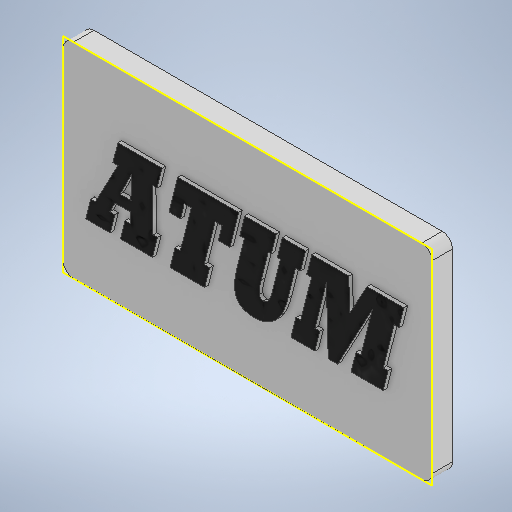
# Autodesk Inventor part: custom plate
Saved by Autodesk Inventor 2025.1 (Build 291241020, 241B)
## iProperties
Created: 2024-12-05
Part Number: custom plate
Material: Generic
Document SubType Name: Modeling
Designer: Hunter Mathis
Density: 1 g/cm^3
Appearance: Default
Author: Hunter Mathis
Autodesk Inventor part; units mm, degrees
ref_plane "YZ Plane" through (0, 0, 0) normal (1, 0, 0) x (0, 1, 0)
ref_plane "XZ Plane" through (0, 0, 0) normal (0, 1, 0) x (-1, 0, 0)
ref_plane "XY Plane" through (0, 0, 0) normal (0, 0, 1) x (1, 0, 0)
sketch "Sketch1" plane through (0, 0, 0) normal (0, 0, 1) x (1, 0, 0)
  line L0 (0, 0) -> (-114.3, 0)
  line L1 (-114.3, 0) -> (-114.3, 63.5)
  line L2 (-114.3, 63.5) -> (0, 63.5)
  line L3 (0, 63.5) -> (0, 0)
  dimension "d7" = 114.3
  dimension "d8" = 63.5
  constraints: 8 end point, 2 parallel, 1 horizontal, 1 perpendicular
  measures "d7" distance of L1.end L2.end
  measures "d8" distance of L0.end L1.end
extrude "Extrusion1" add sketch "Sketch1" along normal blind 6.35
sketch "Sketch2" plane through (0, 0, 6.35) normal (0, 0, 1) x (1, 0, 0)
  line L0 (0, 0) -> (0, 63.5) projected
  line L1 (-114.3, 63.5) -> (-114.3, 0) projected
  line L2 (-114.3, 0) -> (0, 0) projected
  line L3 (0, 63.5) -> (-114.3, 63.5) projected
sketch "Sketch3" plane through (0, 0, 6.35) normal (0, 0, 1) x (1, 0, 0)
  line L0 (-106.4932, 35.0591) -> (-47.8221, 35.0591) construction
  line L1 (-47.8221, 35.0591) -> (-47.8221, 28.1142) construction
  line L2 (-47.8221, 28.1142) -> (-106.4932, 28.1142) construction
  line L3 (-106.4932, 28.1142) -> (-106.4932, 35.0591) construction
  line L4 (-114.3, 63.5) -> (-114.3, 0) projected
  line L5 (-98.6267, 19.0903) -> (-106.1716, 19.0903)
  line L6 (-106.1716, 19.0903) -> (-104.6284, 25.1777)
  line L7 (-104.6284, 25.1777) -> (-103.1708, 25.1777)
  line L8 (-103.1708, 25.1777) -> (-96.226, 38.4029)
  line L9 (-96.226, 38.4029) -> (-97.7693, 38.4029)
  line L10 (-97.7693, 38.4029) -> (-96.2046, 44.4903)
  line L11 (-96.2046, 44.4903) -> (-82.5293, 44.4903)
  line L12 (-82.5293, 44.4903) -> (-84.094, 38.4029)
  line L13 (-84.094, 38.4029) -> (-85.6159, 38.4029)
  line L14 (-85.6159, 38.4029) -> (-85.3587, 25.1777)
  line L15 (-85.3587, 25.1777) -> (-83.9654, 25.1777)
  line L16 (-83.9654, 25.1777) -> (-85.5087, 19.0903)
  line L17 (-85.5087, 19.0903) -> (-95.4329, 19.0903)
  line L18 (-95.4329, 19.0903) -> (-94.0182, 24.6633)
  line L19 (-94.0182, 24.6633) -> (-92.3463, 24.6633)
  line L20 (-92.3463, 24.6633) -> (-92.2606, 27.857)
  line L21 (-92.2606, 27.857) -> (-97.1262, 27.857)
  line L22 (-97.1262, 27.857) -> (-98.7767, 24.6633)
  line L23 (-98.7767, 24.6633) -> (-97.212, 24.6633)
  line L24 (-97.212, 24.6633) -> (-98.6267, 19.0903)
  line L25 (-92.0248, 38.0385) -> (-95.6044, 31.0079)
  line L26 (-95.6044, 31.0079) -> (-92.1963, 31.0079)
  line L27 (-92.1963, 31.0079) -> (-92.0248, 38.0385)
  line L28 (-69.3256, 19.0903) -> (-80.0429, 19.0903)
  line L29 (-80.0429, 19.0903) -> (-78.4781, 25.1777)
  line L30 (-78.4781, 25.1777) -> (-76.8491, 25.1777)
  line L31 (-76.8491, 25.1777) -> (-73.4625, 38.4029)
  line L32 (-73.4625, 38.4029) -> (-75.6702, 38.4029)
  line L33 (-75.6702, 38.4029) -> (-76.8277, 33.7944)
  line L34 (-76.8277, 33.7944) -> (-80.4073, 33.7944)
  line L35 (-80.4073, 33.7944) -> (-77.6851, 44.4903)
  line L36 (-77.6851, 44.4903) -> (-58.8012, 44.4903)
  line L37 (-58.8012, 44.4903) -> (-61.5234, 33.7944)
  line L38 (-61.5234, 33.7944) -> (-65.103, 33.7944)
  line L39 (-65.103, 33.7944) -> (-63.9241, 38.4029)
  line L40 (-63.9241, 38.4029) -> (-66.0889, 38.4029)
  line L41 (-66.0889, 38.4029) -> (-69.4756, 25.1777)
  line L42 (-69.4756, 25.1777) -> (-67.7823, 25.1777)
  line L43 (-67.7823, 25.1777) -> (-69.3256, 19.0903)
  line L44 (-56.9792, 38.4029) -> (-58.4368, 38.4029)
  line L45 (-58.4368, 38.4029) -> (-56.8935, 44.4903)
  line L46 (-56.8935, 44.4903) -> (-47.1622, 44.4903)
  line L47 (-47.1622, 44.4903) -> (-48.7055, 38.4029)
  line L48 (-48.7055, 38.4029) -> (-49.6272, 38.4029)
  line L49 (-49.6272, 38.4029) -> (-51.7921, 29.829)
  spline S0 degree 2 poles (-51.7921, 29.829) (-52.5852, 26.7639) (-52.4351, 25.6493) knots 0 0 0 1 1 1
  spline S1 degree 2 poles (-52.4351, 25.6493) (-52.2636, 24.5561) (-51.1276, 24.5561) knots 0 0 0 1 1 1
  spline S2 degree 2 poles (-51.1276, 24.5561) (-50.1845, 24.5561) (-49.5414, 25.4778) knots 0 0 0 1 1 1
  spline S3 degree 2 poles (-49.5414, 25.4778) (-48.877, 26.3995) (-48.1482, 29.2289) knots 0 0 0 1 1 1
  line L50 (-48.1482, 29.2289) -> (-45.8118, 38.4029)
  line L51 (-45.8118, 38.4029) -> (-46.7764, 38.4029)
  line L52 (-46.7764, 38.4029) -> (-45.2331, 44.4903)
  line L53 (-45.2331, 44.4903) -> (-38.0739, 44.4903)
  line L54 (-38.0739, 44.4903) -> (-39.6172, 38.4029)
  line L55 (-39.6172, 38.4029) -> (-41.1391, 38.4029)
  line L56 (-41.1391, 38.4029) -> (-43.4754, 29.2074)
  spline S4 degree 2 poles (-43.4754, 29.2074) (-44.3757, 25.6707) (-45.7046, 23.4201) knots 0 0 0 1 1 1
  spline S5 degree 2 poles (-45.7046, 23.4201) (-47.0336, 21.2123) (-49.1342, 19.9477) knots 0 0 0 1 1 1
  spline S6 degree 2 poles (-49.1342, 19.9477) (-51.2348, 18.683) (-53.8284, 18.683) knots 0 0 0 1 1 1
  spline S7 degree 2 poles (-53.8284, 18.683) (-55.9289, 18.683) (-57.3651, 19.3475) knots 0 0 0 1 1 1
  spline S8 degree 2 poles (-57.3651, 19.3475) (-58.8441, 20.012) (-59.4442, 21.3624) knots 0 0 0 1 1 1
  spline S9 degree 2 poles (-59.4442, 21.3624) (-60.0658, 22.6913) (-60.0444, 24.599) knots 0 0 0 1 1 1
  spline S10 degree 2 poles (-60.0444, 24.599) (-60.023, 26.4424) (-59.0584, 30.2577) knots 0 0 0 1 1 1
  line L57 (-59.0584, 30.2577) -> (-56.9792, 38.4029)
  line L58 (-35.1803, 19.0903) -> (-42.5538, 19.0903)
  line L59 (-42.5538, 19.0903) -> (-41.0105, 25.1777)
  line L60 (-41.0105, 25.1777) -> (-39.5529, 25.1777)
  line L61 (-39.5529, 25.1777) -> (-36.1662, 38.4029)
  line L62 (-36.1662, 38.4029) -> (-37.6667, 38.4029)
  line L63 (-37.6667, 38.4029) -> (-36.1234, 44.4903)
  line L64 (-36.1234, 44.4903) -> (-24.6559, 44.4903)
  line L65 (-24.6559, 44.4903) -> (-24.3344, 34.6732)
  line L66 (-24.3344, 34.6732) -> (-18.9757, 44.4903)
  line L67 (-18.9757, 44.4903) -> (-7.5511, 44.4903)
  line L68 (-7.5511, 44.4903) -> (-9.0944, 38.4029)
  line L69 (-9.0944, 38.4029) -> (-10.5948, 38.4029)
  line L70 (-10.5948, 38.4029) -> (-13.96, 25.1777)
  line L71 (-13.96, 25.1777) -> (-12.4381, 25.1777)
  line L72 (-12.4381, 25.1777) -> (-13.9814, 19.0903)
  line L73 (-13.9814, 19.0903) -> (-23.9271, 19.0903)
  line L74 (-23.9271, 19.0903) -> (-22.3624, 25.1777)
  line L75 (-22.3624, 25.1777) -> (-20.8405, 25.1777)
  line L76 (-20.8405, 25.1777) -> (-17.2395, 39.346)
  line L77 (-17.2395, 39.346) -> (-28.1497, 19.0903)
  line L78 (-28.1497, 19.0903) -> (-31.0005, 19.0903)
  line L79 (-31.0005, 19.0903) -> (-31.5792, 39.1745)
  line L80 (-31.5792, 39.1745) -> (-35.1374, 25.1777)
  line L81 (-35.1374, 25.1777) -> (-33.637, 25.1777)
  line L82 (-33.637, 25.1777) -> (-35.1803, 19.0903)
  point P0 (0, 0)
  constraints: 2 other
extrude "Extrusion2" add sketch "Sketch3" along normal blind 1.143
fillet "Fillet2" radius 3.175 4 edges at (-114.3, 63.5, 3.175) (-114.3, 0, 3.175) (0, 0, 3.175) (0, 63.5, 3.175)
body "Solid1"
